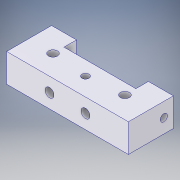
# Autodesk Inventor part: exBase
Saved by Autodesk Inventor 2017 (Build 210142000, 142)
## iProperties
Created: 2017-03-10
Part Number: exBase
Material: Generic
Document SubType Name: Modeling
Designer: Naga
Density: 1 g/cm^3
Appearance: Cool White
Author: Naga
Autodesk Inventor part; units mm, degrees
ref_plane "YZ Plane" through (0, 0, 0) normal (1, 0, 0) x (0, 1, 0)
ref_plane "XZ Plane" through (0, 0, 0) normal (0, 1, 0) x (-1, 0, 0)
ref_plane "XY Plane" through (0, 0, 0) normal (0, 0, 1) x (1, 0, 0)
sketch "Sketch1" plane through (0, 0, 0) normal (0, 1, 0) x (-1, 0, 0)
  line L0 (0, 0) -> (43, 0)
  line L1 (43, 0) -> (43, -61)
  line L2 (43, -61) -> (0, -61)
  line L3 (0, -61) -> (0, 0)
  dimension "d0" = 61
  dimension "d1" = 43
  constraints: 8 end point, 2 parallel, 1 horizontal, 1 perpendicular
  measures "d0" distance of L0.end L1.end
  measures "d1" distance of L1.end L2.end
extrude "Extrusion1" add sketch "Sketch1" along normal blind 10
sketch "Sketch2" plane through (0, 0, 0) normal (1, 0, 0) x (0, 0, -1)
  line L0 (0, 0) -> (0, 10) projected
  line L1 (0, 5) -> (12.5, 5)
  circle A0 centre (12.5, 5) radius 1.25
  line L2 (0, 10) -> (61, 10) projected
  line L3 (30.5, 10) -> (30.5, 0)
  circle A1 centre (48.5, 5) radius 1.25
  dimension "d4" = 12.5
  dimension "d5" = 2.5
  constraints: 4 end point, 2 centre point, 2 midpoint, 1 coincident, 1 horizontal, 1 symmetric about line, 1 vertical, 1 other
  measures "d4" distance of L1.start L1.end
  measures "d5" diameter of A0
extrude "Extrusion2" cut sketch "Sketch2" against normal blind 5
sketch "Sketch3" plane through (-43, 0, -61) normal (-1, 0, 0) x (0, 0, 1)
  line L0 (61, 0) -> (0, 0) projected
  line L1 (61, 0) -> (61, 10) projected
  line L2 (0, 10) -> (61, 10) projected
  line L3 (0, 0) -> (0, 10) projected
  circle A0 centre (48.5, 5) radius 1.25 projected
  circle A1 centre (12.5, 5) radius 1.25 projected
extrude "Extrusion3" cut sketch "Sketch3" against normal blind 5 contours A0 | A1
sketch "Sketch4" plane through (0, 10, 0) normal (0, 1, 0) x (1, 0, 0)
  line L0 (-43, 0) -> (0, 0) projected
  line L1 (0, 61) -> (-43, 61) projected
  line L2 (-21.5, 0) -> (-21.5, 6.35)
  line L3 (-21.5, 61) -> (-21.5, 54.65)
  circle A0 centre (-21.5, 6.35) radius 1.25
  circle A1 centre (-21.5, 54.65) radius 1.25
  dimension "d10" = 6.35
  dimension "d11" = 6.35
  dimension "d12" = 2.5
  dimension "d13" = 2.5
  constraints: 4 end point, 2 centre point, 2 coincident, 2 midpoint, 2 vertical
  measures "d10" distance of L2.start L2.end
  measures "d11" distance of L3.start L3.end
  measures "d12" diameter of A0
  measures "d13" diameter of A1
extrude "Extrusion4" cut sketch "Sketch4" against normal up to surface (10 mm away)
sketch "Sketch5" plane through (0, 10, 0) normal (0, 1, 0) x (1, 0, 0)
  circle A0 centre (-21.5, 6.35) radius 1.25 projected
  circle A1 centre (-21.5, 54.65) radius 1.25 projected
  line L0 (-43, 0) -> (0, 0) projected
  line L1 (0, 0) -> (0, 61) projected
  line L2 (0, 61) -> (-43, 61) projected
  line L3 (-43, 61) -> (-43, 0) projected
  line L4 (-8.8, 11.45) -> (-34.2, 11.45)
  line L5 (-34.2, 11.45) -> (-34.2, 49.55)
  line L6 (-34.2, 49.55) -> (-8.8, 49.55)
  line L7 (-8.8, 49.55) -> (-8.8, 11.45)
  line L8 (-8.8, 11.45) -> (-34.2, 49.55) construction
  line L9 (-34.2, 11.45) -> (-8.8, 49.55) construction
  point P0 (-21.5, 30.5)
  dimension "d16" = 25.4
  dimension "d17" = 38.1
  constraints: 12 end point, 2 midpoint, 2 parallel, 1 horizontal, 1 perpendicular
  measures "d16" distance of L5.end L6.end
  measures "d17" distance of L4.end L5.end
extrude "Extrusion5" cut sketch "Sketch5" against normal up to surface (10 mm away) contours L4 L5 L6 L7
sketch "Sketch6" plane through (0, 0, 0) normal (1, 0, 0) x (0, 0, -1)
  line L0 (0, 0) -> (0, 10) projected
  line L1 (61, 0) -> (0, 0) projected
  line L2 (0, 10) -> (15.875, 10)
  line L3 (15.875, 10) -> (15.875, 0)
  line L4 (15.875, 0) -> (0, 0)
  line L5 (0, 0) -> (0, 10)
  circle A0 centre (12.5, 5) radius 1.25 projected
  circle A1 centre (48.5, 5) radius 1.25 projected
  line L6 (61, 0) -> (0, 0) projected
  line L7 (61, 0) -> (61, 10) projected
  line L8 (0, 10) -> (61, 10) projected
  line L9 (0, 0) -> (0, 10) projected
  dimension "d20" = 15.875
  constraints: 8 end point, 2 parallel, 1 horizontal, 1 perpendicular, 1 point on line
  measures "d20" distance of L3.end L4.end
extrude "Extrusion6" cut sketch "Sketch6" against normal up to surface (43 mm away) contours L3 L8 L7 L1 | A1
sketch "Sketch7" plane through (0, 10, 0) normal (0, 1, 0) x (1, 0, 0)
  line L0 (-34.2, 15.875) -> (-43, 15.875) projected
  line L1 (-43, 15.875) -> (-43, 0) projected
  line L2 (-43, 0) -> (0, 0) projected
  line L3 (0, 0) -> (0, 15.875) projected
  line L4 (0, 15.875) -> (-8.8, 15.875) projected
  line L5 (-8.8, 15.875) -> (-8.8, 11.45) projected
  line L6 (-8.8, 11.45) -> (-34.2, 11.45) projected
  line L7 (-34.2, 11.45) -> (-34.2, 15.875) projected
  circle A0 centre (-21.5, 6.35) radius 1.25 projected
  line L8 (-43, 0) -> (0, 0) projected
  line L9 (-21.5, 0) -> (-34.2, 0)
  line L10 (-34.2, 0) -> (-34.2, 7.5692)
  circle A1 centre (-34.2, 7.5692) radius 1.5875
  line L11 (-21.5, 0) -> (-21.5, 3.1877)
  circle A2 centre (-8.8, 7.5692) radius 1.5875
  dimension "d23" = 12.7
  dimension "d24" = 7.5692
  dimension "d25" = 3.175
  constraints: 6 end point, 2 centre point, 1 coincident, 1 midpoint, 1 perpendicular, 1 point on line, 1 symmetric about line, 1 vertical, 1 other
  measures "d23" distance of L9.start L9.end
  measures "d24" distance of L9.end L10.end
  measures "d25" diameter of A1
extrude "Extrusion7" cut sketch "Sketch7" against normal blind 25.4 contours A1 | A2
sketch "Sketch8" plane through (0, 0, -15.875) normal (0, 0, -1) x (-1, 0, 0)
  line L0 (34.2, 0) -> (8.8, 0) projected
  line L1 (8.8, 10) -> (34.2, 10) projected
  line L2 (8.8, 10) -> (8.8, 0) projected
  line L3 (0, 0) -> (43, 0) projected
  line L4 (8.8, 10) -> (15.15, 10)
  line L5 (15.15, 10) -> (15.15, 0)
  line L6 (15.15, 0) -> (8.8, 0)
  line L7 (8.8, 0) -> (8.8, 10)
  circle A0 centre (15.15, 5) radius 1.5875
  line L8 (34.2, 10) -> (27.85, 10)
  line L9 (27.85, 10) -> (27.85, 0)
  line L10 (27.85, 0) -> (34.2, 0)
  line L11 (34.2, 0) -> (34.2, 10)
  circle A1 centre (27.85, 5) radius 1.5875
  line L12 (34.2, 10) -> (34.2, 0) projected
  line L13 (8.8, 10) -> (8.8, 0) projected
  dimension "d28" = 6.35
  dimension "d29" = 3.175
  dimension "d30" = 6.35
  dimension "d31" = 3.175
  constraints: 16 end point, 4 parallel, 2 centre point, 2 horizontal, 2 midpoint, 2 perpendicular, 2 point on line
  measures "d28" distance of L5.end L6.end
  measures "d29" diameter of A0
  measures "d30" distance of L10.end L9.end
  measures "d31" diameter of A1
extrude "Extrusion8" cut sketch "Sketch8" against normal up to surface (15.875 mm away) contours A1 L9 | L9 A1 | A0 L5 | L5 A0
body "Solid1"
